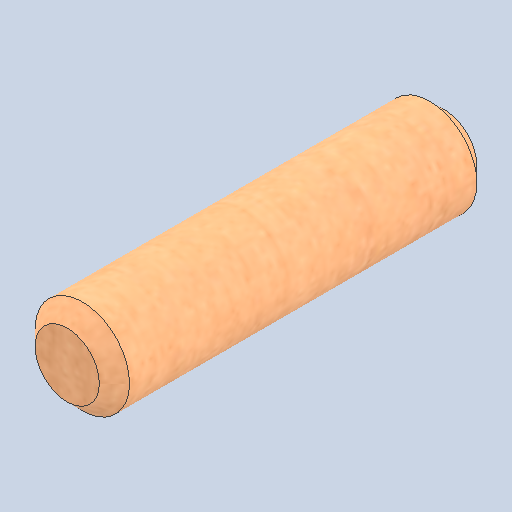
# Autodesk Inventor part: hex axle pin
Saved by Autodesk Inventor 2024 (Build 280153000, 153)
## iProperties
Created: 2023-05-28
Part Number: hex axle pin
Material: Generic
Document SubType Name: Modeling
Designer: _Astitva_Aryan_
Density: 1 g/cm^3
Appearance: Default
Author: _Astitva_Aryan_
Autodesk Inventor part; units mm, degrees
ref_plane "YZ Plane" through (0, 0, 0) normal (1, 0, 0) x (0, 1, 0)
ref_plane "XZ Plane" through (0, 0, 0) normal (0, 1, 0) x (-1, 0, 0)
ref_plane "XY Plane" through (0, 0, 0) normal (0, 0, 1) x (1, 0, 0)
sketch "Sketch1" plane through (0, 0, 0) normal (0, 0, 1) x (1, 0, 0)
  circle A0 centre (0, 0) radius 1.1906
  dimension "d0" = 2.3813
  constraints: 1 centre point, 1 coincident
  measures "d0" diameter of A0
extrude "Extrusion1" add sketch "Sketch1" along normal mid plane 9.525
chamfer "Chamfer1" distance 0.381 angle 45 2 edges at (-1.1906, 0, -4.7625) (-1.1906, 0, 4.7625)
scale "Scale1" factors (10, 10, 10) then translate (0, 0, 0) bodies 1
body "Solid1"
